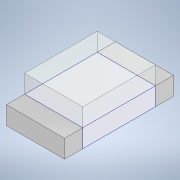
# Autodesk Inventor part: Led_0603
Saved by Autodesk Inventor 2020 (Build 240168000, 168)
## iProperties
Created: 2020-01-12
Part Number: Led_0603
Material: Generic
Document SubType Name: Modeling
Designer: ermoz
Density: 1 g/cm^3
Appearance: Default
Author: ermoz
Autodesk Inventor part; units mm, degrees
ref_plane "YZ Plane" through (0, 0, 0) normal (1, 0, 0) x (0, 1, 0)
ref_plane "XZ Plane" through (0, 0, 0) normal (0, 1, 0) x (-1, 0, 0)
ref_plane "XY Plane" through (0, 0, 0) normal (0, 0, 1) x (1, 0, 0)
sketch "Sketch1" plane through (0, 0, 0) normal (0, 1, 0) x (-1, 0, 0)
  line L0 (-0.4, 0.75) -> (0.4, 0.75)
  line L1 (0.4, 0.75) -> (0.4, -0.75)
  line L2 (0.4, -0.75) -> (-0.4, -0.75)
  line L3 (-0.4, -0.75) -> (-0.4, 0.75)
  line L4 (-0.4, 0.75) -> (0.4, -0.75) construction
  line L5 (0.4, 0.75) -> (-0.4, -0.75) construction
  point P0 (0, 0)
  dimension "d0" = 0.8
  dimension "d1" = 1.5
  constraints: 12 end point, 2 midpoint, 2 parallel, 1 horizontal, 1 perpendicular
  measures "d0" distance of L1.end L2.end
  measures "d1" distance of L0.end L1.end
extrude "Extrusion1" add sketch "Sketch1" along normal blind 0.5
sketch "Sketch2" plane through (0, 0.5, 0) normal (0, 1, 0) x (1, 0, 0)
  line L0 (0.4, -0.5) -> (-0.4, -0.5)
  line L1 (-0.4, -0.5) -> (0.4, -0.5)
  line L2 (0.4, -0.75) -> (0.4, 0.75) projected
  line L3 (-0.4, -0.5) -> (0.4, -0.5)
  line L4 (0.4, -0.5) -> (0.4, 0.5)
  line L5 (0.4, 0.5) -> (-0.4, 0.5)
  line L6 (-0.4, 0.5) -> (-0.4, -0.5)
  point P0 (0, 0)
  point P1 (-0.4, 0.75)
  point P2 (-0.4, -0.75)
  dimension "d6" = 1
  constraints: 12 end point, 2 horizontal, 2 parallel, 1 perpendicular, 1 point on line
  measures "d6" distance of L4.end L3.end
split body "Split1" sketch "Sketch2" result two bodies curves L4 L5 L6 L3 first body at (0.1333, 0.1, 0.1667)
sketch "Sketch3" plane through (0, 0.5, 0) normal (0, 1, 0) x (1, 0, 0)
  line L0 (-0.8884, -1.0057) -> (0.9425, -1.0057)
  line L1 (0.9425, -1.0057) -> (0.9425, 1.4927)
  line L2 (0.9425, 1.4927) -> (-0.8884, 1.4927)
  line L3 (-0.8884, 1.4927) -> (-0.8884, -1.0057)
  point P0 (0, 0)
  constraints: 8 end point, 2 parallel, 1 horizontal, 1 perpendicular
extrude "Extrusion2" cut sketch "Sketch3" against normal blind 0.25 bodies 3
sketch "Sketch4" plane through (0.4, 0, 0.5) normal (1, 0, 0) x (0, 0, -1)
  line L0 (0, 0.5) -> (0, 0) projected
  line L1 (1, 0.5) -> (1, 0) projected
  line L2 (0, 0.25) -> (1, 0.25)
  line L3 (1, 0.25) -> (1, 0)
  line L4 (1, 0) -> (0, 0)
  line L5 (0, 0) -> (0, 0.25)
  point P0 (0.5, 0)
  constraints: 8 end point, 2 parallel, 1 horizontal, 1 midpoint, 1 perpendicular
split body "Split2" sketch "Sketch4" result two bodies bodies 2 curves L2 L3 L4 L5 first body at (0.1333, 0.4, 0.1667)
body "Solid3"
body "Solid4"
body "Solid5"
